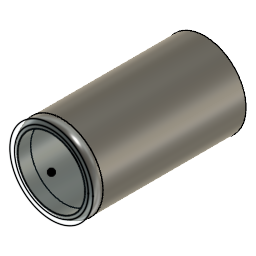
ACOPLE_RUEDA_PILAR (Autodesk Fusion 360 design; units mm, degrees)
Autodesk Fusion 360 part; units mm, degrees
sketch "Boceto1" plane through (0, 0, 0) normal (0, 1, 0) x (1, 0, 0)
  circle A0 centre (0, 0) radius 8
  circle A1 centre (0, 0) radius 7.1
  circle A2 centre (0, 0) radius 6.5
  dimension "d1" = 16
  dimension "d2" = 14.2
  dimension "d3" = 13
  constraint coincident A0.centre A1.centre
  constraint concentric A0 A1
  measures "d1" diameter of A0
  measures "d2" diameter of A1
  measures "d3" diameter of A2
extrude "Extruir1" add sketch "Boceto1" along normal blind 29.5 contours A0
extrude "Extruir4" add sketch "Boceto1" along normal blind 2.5 contours A1
fillet "Empalme1" radius 2 1 edges at (-7.4586, 0, 2.8929)
